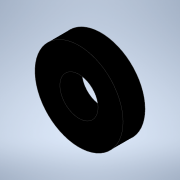
# Autodesk Inventor part: UUW-0512-30BH
Saved by Autodesk Inventor 2022.3 (Build 263350000, 350)
## iProperties
Part Number: UUW-0512-30BH
Material: ステンレス鋼 AISI 304
Document SubType Name: Modeling
Designer: Masato Kubotera
Density: 7.2286 g/cm^3
Appearance: 陽極酸化 - 黒
Mass: 0.7594 g
Surface Area: 2.57862 cm^2
Volume: 0.105055 cm^3
Description: ReadyMade
Catalog Web Link: https://www.hirosugi-net.co.jp/shop/g/g59042/
Author: Masato Kubotera
Autodesk Inventor part; units mm, degrees
ref_plane "YZ Plane" through (0, 0, 0) normal (1, 0, 0) x (0, 1, 0)
ref_plane "XZ Plane" through (0, 0, 0) normal (0, 1, 0) x (-1, 0, 0)
ref_plane "XY Plane" through (0, 0, 0) normal (0, 0, 1) x (1, 0, 0)
sketch "スケッチ1" plane through (0, 0, 0) normal (0, 0, 1) x (1, 0, 0)
  circle A0 centre (0, 0) radius 2.6
  circle A1 centre (0, 0) radius 6
  dimension "d0" = 5.2
  dimension "d1" = 12
  constraints: 2 centre point, 2 coincident
  measures "d0" diameter of A0
  measures "d1" diameter of A1
extrude "押し出し1" add sketch "スケッチ1" along normal blind 3
